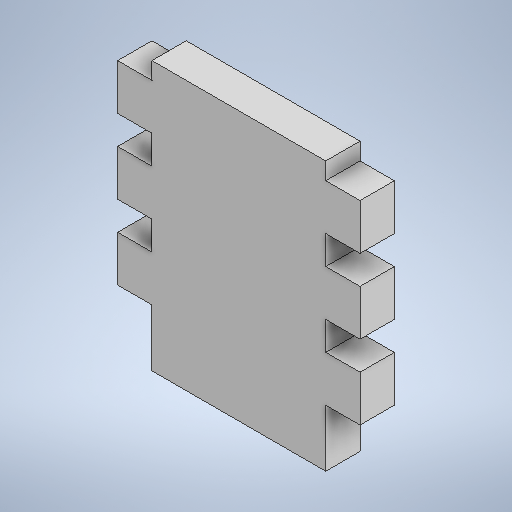
# Autodesk Inventor part: sort support V2 wall 2
Saved by Autodesk Inventor 2025.3 (Build 293356000, 356)
## iProperties
Created: 2026-04-30
Part Number: sort support V2 wall 2
Material: Generic
Document SubType Name: Modeling
Designer: kamal
Density: 1 g/cm^3
Appearance: Default
Author: kamal
Autodesk Inventor part; units mm, degrees
ref_plane "YZ Plane" through (0, 0, 0) normal (1, 0, 0) x (0, 1, 0)
ref_plane "XZ Plane" through (0, 0, 0) normal (0, 1, 0) x (-1, 0, 0)
ref_plane "XY Plane" through (0, 0, 0) normal (0, 0, 1) x (1, 0, 0)
sketch "Sketch1" plane through (0, 0, 0) normal (0, 0, 1) x (1, 0, 0)
  line L0 (0, 0) -> (0, 10)
  line L1 (0, 10) -> (6, 10)
  line L2 (6, 10) -> (6, 18)
  line L3 (6, 18) -> (0, 18)
  line L4 (0, 18) -> (0, 23)
  line L5 (0, 23) -> (6, 23)
  line L6 (6, 23) -> (6, 31)
  line L7 (6, 31) -> (0, 31)
  line L8 (0, 31) -> (0, 36)
  line L9 (0, 36) -> (6, 36)
  line L10 (6, 36) -> (6, 44)
  line L11 (6, 44) -> (0, 44)
  line L12 (0, 44) -> (0, 47)
  line L13 (0, 47) -> (-15.2, 47)
  line L14 (-15.2, 47) -> (-15.2, 0) construction
  line L15 (-15.2, 0) -> (0, 0)
  line L16 (-30.4, 0) -> (-30.4, 10)
  line L17 (-30.4, 10) -> (-36.4, 10)
  line L18 (-36.4, 10) -> (-36.4, 18)
  line L19 (-36.4, 18) -> (-30.4, 18)
  line L20 (-30.4, 18) -> (-30.4, 23)
  line L21 (-30.4, 23) -> (-36.4, 23)
  line L22 (-36.4, 23) -> (-36.4, 31)
  line L23 (-36.4, 31) -> (-30.4, 31)
  line L24 (-30.4, 31) -> (-30.4, 36)
  line L25 (-30.4, 36) -> (-36.4, 36)
  line L26 (-36.4, 36) -> (-36.4, 44)
  line L27 (-36.4, 44) -> (-30.4, 44)
  line L28 (-30.4, 44) -> (-30.4, 47)
  line L29 (-30.4, 47) -> (-15.2, 47)
  line L30 (-15.2, 0) -> (-30.4, 0)
  dimension "d30" = 10
  dimension "d31" = 6
  dimension "d32" = 8
  dimension "d33" = 5
  dimension "d34" = 8
  dimension "d35" = 5
  dimension "d36" = 6
  dimension "d37" = 8
  dimension "d38" = 6
  dimension "d39" = 3
  dimension "d40" = 15.2
  constraints: 62 end point, 20 point on line, 14 symmetric about line, 7 perpendicular, 1 horizontal, 1 vertical
  measures "d30" distance of L0.start L0.end
  measures "d31" distance of L0.end L1.end
  measures "d32" distance of L1.end L2.end
  measures "d33" distance of L3.end L4.end
  measures "d34" distance of L5.end L6.end
  measures "d35" distance of L7.end L8.end
  measures "d36" distance of L8.end L9.end
  measures "d37" distance of L9.end L10.end
  measures "d38" distance of L10.end L11.end
  measures "d39" distance of L11.end L12.end
  measures "d40" distance of L12.end L13.end
extrude "Extrusion1" add sketch "Sketch1" along normal blind 6
body "Solid1"
